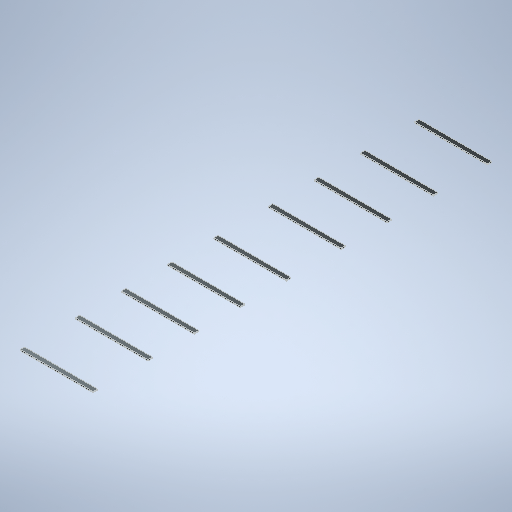
# Autodesk Inventor part: Cross Supports
Saved by Autodesk Inventor 2025 (Build 290162000, 162)
## iProperties
Created: 2024-06-26
Part Number: Cross Supports
Material: Iron, Cast
Document SubType Name: Modeling
Designer: track
Density: 7.15 g/cm^3
Appearance: Iron Gray
Author: track
Autodesk Inventor part; units mm, degrees
ref_plane "YZ Plane" through (0, 0, 0) normal (1, 0, 0) x (0, 1, 0)
ref_plane "XZ Plane" through (0, 0, 0) normal (0, 1, 0) x (-1, 0, 0)
ref_plane "XY Plane" through (0, 0, 0) normal (0, 0, 1) x (1, 0, 0)
sketch "Sketch1" plane through (838.2, 0, 4876.8) normal (0, 1, 0) x (-1, 0, 0)
  line L0 (1676.4, 0) -> (1676.4, -9753.6)
  line L1 (0, 0) -> (0, -9753.6)
  line L2 (1676.4, -381) -> (0, -381)
  line L3 (0, -381) -> (0, -482.6)
  line L4 (0, -482.6) -> (1676.4, -482.6)
  line L5 (1676.4, -482.6) -> (1676.4, -381)
  line L6 (0, 0) -> (1676.4, 0)
  line L7 (1676.4, -1651) -> (0, -1651)
  line L8 (0, -1651) -> (0, -1752.6)
  line L9 (0, -1752.6) -> (1676.4, -1752.6)
  line L10 (1676.4, -1752.6) -> (1676.4, -1651)
  line L11 (1676.4, -2717.8) -> (0, -2717.8)
  line L12 (0, -2717.8) -> (0, -2819.4)
  line L13 (0, -2819.4) -> (1676.4, -2819.4)
  line L14 (1676.4, -2819.4) -> (1676.4, -2717.8)
  line L15 (1676.4, -3778.25) -> (0, -3778.25)
  line L16 (0, -3778.25) -> (0, -3879.85)
  line L17 (0, -3879.85) -> (1676.4, -3879.85)
  line L18 (1676.4, -3879.85) -> (1676.4, -3778.25)
  line L19 (1676.4, -4841.875) -> (0, -4841.875)
  line L20 (0, -4841.875) -> (0, -4943.475)
  line L21 (0, -4943.475) -> (1676.4, -4943.475)
  line L22 (1676.4, -4943.475) -> (1676.4, -4841.875)
  line L23 (1676.4, -6102.35) -> (0, -6102.35)
  line L24 (0, -6102.35) -> (0, -6203.95)
  line L25 (0, -6203.95) -> (1676.4, -6203.95)
  line L26 (1676.4, -6203.95) -> (1676.4, -6102.35)
  line L27 (1676.4, -7162.8) -> (0, -7162.8)
  line L28 (0, -7162.8) -> (0, -7264.4)
  line L29 (0, -7264.4) -> (1676.4, -7264.4)
  line L30 (1676.4, -7264.4) -> (1676.4, -7162.8)
  line L31 (1676.4, -8331.2) -> (0, -8331.2)
  line L32 (0, -8331.2) -> (0, -8229.6)
  line L33 (0, -8229.6) -> (1676.4, -8229.6)
  line L34 (1676.4, -8229.6) -> (1676.4, -8331.2)
  line L35 (1676.4, -9474.2) -> (0, -9474.2)
  line L36 (0, -9474.2) -> (0, -9575.8)
  line L37 (0, -9575.8) -> (1676.4, -9575.8)
  line L38 (1676.4, -9575.8) -> (1676.4, -9474.2)
  line L39 (1676.4, -9753.6) -> (0, -9753.6)
  point P0 (0, -9474.2)
  point P1 (0, -8331.2)
  point P2 (0, -7162.8)
  point P3 (0, -6102.35)
  point P4 (0, -4841.875)
  point P5 (0, -3778.25)
  point P6 (0, -2717.8)
  point P7 (0, -1651)
  point P8 (0, -381)
  dimension "d16" = 101.6
  dimension "d17" = 381
  dimension "d14" = 101.6
  dimension "d15" = 1168.4
  dimension "d12" = 101.6
  dimension "d10" = 101.6
  dimension "d13" = 965.2
  dimension "d11" = 958.85
  dimension "d8" = 101.6
  dimension "d9" = 962.025
  dimension "d7" = 1158.875
  dimension "d6" = 101.6
  dimension "d5" = 958.85
  dimension "d4" = 101.6
  dimension "d3" = 965.2
  dimension "d1" = 177.8
  dimension "d0" = 101.6
  dimension "d2" = 101.6
  constraints: 76 end point, 18 parallel, 9 horizontal, 9 perpendicular, 24 other
  measures "d16" distance between parallel lines of L2 L4
  measures "d17" distance between parallel lines of L6 L2
  measures "d14" distance between parallel lines of L7 L9
  measures "d15" distance between parallel lines of L7 L4
  measures "d12" distance between parallel lines of L13 L11
  measures "d10" distance between parallel lines of L17 L15
  measures "d13" distance between parallel lines of L9 L11
  measures "d11" distance between parallel lines of L13 L15
  measures "d8" distance between parallel lines of L21 L19
  measures "d9" distance between parallel lines of L17 L19
  measures "d7" distance between parallel lines of L21 L23
  measures "d6" distance between parallel lines of L25 L23
  measures "d5" distance between parallel lines of L25 L27
  measures "d4" distance between parallel lines of L29 L27
  measures "d3" distance between parallel lines of L29 L33
  measures "d1" distance between parallel lines of L39 L37
  measures "d0" distance between parallel lines of L37 L35
  measures "d2" distance between parallel lines of L31 L33
extrude "Extrusion1" add sketch "Sketch1" along normal blind 25.4 contours L0 L4 L1 L2 | L0 L9 L1 L7 | L0 L13 L1 L11 | L0 L17 L1 L15 | L0 L21 L1 L19 | L0 L25 L1 L23 | L0 L29 L1 L27 | L0 L31 L1 L33 | L0 L37 L1 L35
body "Solid1"
